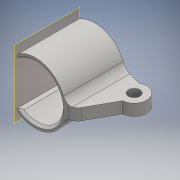
# Autodesk Inventor part: Radio Mic Holder
Saved by Autodesk Inventor 2016 (Build 200138000, 138)
## iProperties
Created: 2019-08-09
Part Number: Radio Mic Holder
Material: Generic
Document SubType Name: Modeling
Designer: DML
Density: 1 g/cm^3
Appearance: Default
Author: DML
Autodesk Inventor part; units mm, degrees
ref_plane "XZ Plane" through (0, 0, 0) normal (0, 1, 0) x (-1, 0, 0)
ref_plane "XY Plane" through (0, 0, 0) normal (0, 0, 1) x (1, 0, 0)
sketch "Sketch1" plane through (0, 0, 0) normal (0, 1, 0) x (-1, 0, 0)
  circle A0 centre (0, 0) radius 17.5
  arc A1 (-20.1304, -3.875) -> (-20.1304, 3.875) centre (0, 0) ccw
  line L0 (-20.5, -3.875) -> (-20.5, -13.4374) construction
  line L1 (-20.5, -13.4374) -> (-20.5, 14.7091) construction
  line L2 (-47.5, 3.875) -> (-47.5, -3.875)
  line L3 (-47.5, -3.875) -> (-20.1304, -3.875)
  line L4 (0, 0) -> (-47.4736, 0) construction
  line L5 (-47.5, 3.875) -> (-20.1304, 3.875)
  dimension "d0" = 35
  dimension "d1" = 3
  dimension "d4" = 27
  constraints: 12 end point, 2 centre point, 2 horizontal, 2 point on circle, 2 point on line, 2 vertical, 1 coincident, 1 perpendicular, 1 tangent
  measures "d0" diameter of A0
  measures "d1" radial gap between concentric circles of A0 A1
  measures "d4" distance of L2.end L0.start
extrude "Extrusion1" add sketch "Sketch1" along normal blind 40
sketch "Sketch2" plane through (20.1304, 0, 3.875) normal (0, 0, 1) x (1, 0, 0)
  line L0 (27.3696, 0) -> (27.3696, 40) projected
  line L1 (2, 40) -> (27.3696, 40)
  line L2 (17.5718, 20.8426) -> (6, 0)
  line L3 (27.3696, 0) -> (0, 0) projected
  line L4 (27.3696, 0) -> (27.3696, 40) projected
  line L5 (6, 0) -> (27.3696, 0)
  line L6 (27.3696, 0) -> (27.3696, 28)
  line L7 (0, 0) -> (0, 40) projected
  arc A0 (17.5718, 20.8426) -> (12.9208, 36.4588) centre (17, 29.173) ccw
  line L8 (12.9208, 36.4588) -> (0, 40)
  circle A1 centre (17, 29.173) radius 3.825
  line L9 (0, 40) -> (27.3696, 40)
  line L10 (27.3696, 0) -> (6, 0)
  point P0 (-20.1304, 0)
  dimension "d10" = 6
  dimension "d14" = 16.7
  dimension "d15" = 17
  dimension "d16" = 7.65
  constraints: 14 end point, 2 centre point, 2 point on circle, 2 point on line, 1 coincident, 1 horizontal, 1 parallel, 1 perpendicular
  measures "d10" distance of L2.end L3.end
  measures "d14" diameter of A0
  measures "d15" distance from line of L7 A0.centre
  measures "d16" diameter of A1
extrude "Extrusion2" cut sketch "Sketch2" against normal blind 40 contours L3 L2 A0 L8 L9 L1 L0 | A1
ref_plane "Work Plane1" through (-12, 0, 0) normal (1, 0, 0) x (0, 1, 0)
split "Split1" plane through (-12, 0, 0) removes the side toward (-1, 0, 0)
chamfer "Chamfer1" distance 1.5 angle 45 1 edges at (17.5, 0, 0)
chamfer "Chamfer2" distance 1.5 angle 45 1 edges at (17.5, 40, 0)
fillet "Fillet1" radius 6 1 edges at (20.1304, 20, 3.875)
fillet "Fillet2" radius 6 1 edges at (20.1304, 20, -3.875)
fillet "Fillet3" radius 6 1 edges at (26.1304, 0, 0)
fillet "Fillet4" radius 3 2 edges at (-12, 20, -16.6208) (-12, 20, 16.6208)
fillet_without_effect "Fillet5"
fillet "Fillet6" radius 3 2 edges at (-12, 20, -12.7377) (-12, 20, 12.7377)
body "Solid1"
